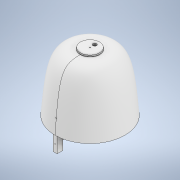
# Autodesk Inventor part: EnclosingRevolver
Saved by Autodesk Inventor 2021.1 (Build 251245010, 245A)
## iProperties
Created: 2023-07-02
Part Number: EnclosingRevolver
Material: ABS Plastic
Document SubType Name: Modeling
Designer: Drake
Density: 1.06 g/cm^3
Appearance: Smooth - White
Author: Drake
Autodesk Inventor part; units mm, degrees
ref_plane "XZ Plane" through (0, 0, 0) normal (0, 1, 0) x (-1, 0, 0)
sketch "Sketch1" plane through (0, 0, 0) normal (0, 1, 0) x (-1, 0, 0)
  circle A0 centre (0, 0) radius 1
  circle A1 centre (0, 0) radius 25
  dimension "d0" = 2
  dimension "d1" = 50
  constraints: 2 centre point, 2 coincident
  measures "d0" diameter of A0
  measures "d1" diameter of A1
extrude "Extrusion1" add sketch "Sketch1" along normal blind 3.7
ref_plane "Work Plane2" through (-25, 0, 0) normal (1, 0, 0) x (0, 1, 0)
ref_plane "Work Plane1" through (25, 0, 0) normal (1, 0, 0) x (0, 1, 0)
sketch "Sketch3" plane through (0, 0, 0) normal (1, 0, 0) x (0, 1, 0)
  line L0 (0, 25.8902) -> (0, 82.1004) construction
  line L1 (0, 82.1004) -> (-19.2329, 82.1004) construction
  line L2 (-19.2329, 82.1004) -> (-150.2459, 92.0453) construction
  line L3 (-150.2459, 92.0453) -> (-151.1107, 92.0453) construction
  spline S0 degree 4 poles (0, 25.8902) (0, 82.1004) (-19.2329, 82.1004) (-150.2459, 92.0453) (-151.1107, 92.0453) knots 1 1 1 1 1 2 2 2 2 2
  line L4 (0, -25) -> (0, 25) projected
  line L5 (-151.1107, 92.0453) -> (-151.1107, 77.0453)
  line L6 (-151.1107, 77.0453) -> (-80.8125, 71.4468) construction
  line L7 (-80.8125, 71.4468) -> (-20.5383, 53.8321) construction
  line L8 (-20.5383, 53.8321) -> (-22.6717, 53.8321) construction
  line L9 (-22.6717, 53.8321) -> (-15, 0) construction
  spline S1 degree 4 poles (-151.1107, 77.0453) (-80.8125, 71.4468) (-20.5383, 53.8321) (-22.6717, 53.8321) (-15, 0) knots 1 1 1 1 1 2 2 2 2 2
  line L10 (0, 25) -> (0, 0)
  line L11 (0, 25) -> (0, 0)
  line L12 (-15, -28.9058) -> (-15, -27.5917)
  line L13 (0, 25.8902) -> (0, -27.5917)
  line L14 (-15, 0) -> (0, 0)
  dimension "d9" = 15
  dimension "d10" = 15
  constraints: 12 end point, 3 horizontal, 2 point on line, 2 vertical, 1 collinear, 1 parallel, 6 other
  measures "d9" distance of L10.end L9.end
  measures "d10" distance of L3.end L5.end
revolve "Revolution1" add sketch "Sketch3" angle 360 about axis through (0, -15, 0) along (0, -1, 0)
mirror "Mirror1" about plane through (0, 0, 0) normal (0, 0, 1) of "Revolution1"
ref_plane "Work Plane3" through (0, 0, 92.0455) normal (0, 0, 1) x (1, 0, 0)
sketch "Sketch4" plane through (0, 0, 92.0455) normal (0, 0, 1) x (1, 0, 0)
  line L0 (-92.0453, -151.1107) -> (92.0453, -151.1107) projected
  line L1 (-92.0453, -151.1107) -> (-92.0453, -139.1107)
  line L2 (-92.0453, -151.1107) -> (-92.0453, -118.1107)
  line L3 (-92.0453, -118.1107) -> (-92.0453, -113.1107)
  line L4 (-92.0453, -113.1107) -> (0, -113.1107)
  point P0 (0, 0)
  point P1 (0, -151.1107)
  dimension "motorwidth" = 12
  dimension "motorlength" = 33
  dimension "allowance" = 5
  constraints: 8 end point, 3 vertical, 1 coincident, 1 perpendicular
  measures "motorwidth" distance of L0.start L1.end
  measures "motorlength" distance of L0.start L2.end
  measures "allowance" distance of L2.end L3.end
hole "Hole1" at (0, -113.1107, 92.0455) direction (0, 0, -1) diameter 3 end through all
thread "Thread1" size "M3x0.5" class "6H" standard "ANSI Metric M Profile" full length
sketch "Sketch5" plane through (0, 3.7, 0) normal (0, 1, 0) x (1, 0, 0)
  point P0 (0, 0)
  point P1 (0.766, -0.6428)
hole "Hole2" at (0.766, 3.7, 0.6428) direction (0, -1, 0) diameter 2 end through all
sketch "Sketch6" plane through (0, -151.1107, 0) normal (0, -1, 0) x (1, 0, 0)
  line L0 (-4.9974, -76.883) -> (-4.9974, -91.9095)
  circle A0 centre (0, 0) radius 92.0453 projected
  line L1 (4.9974, -91.9095) -> (4.9974, -76.883)
  circle A1 centre (0, 0) radius 77.0453
  point P0 (0, 77.0453)
  point P1 (0, 92.0453)
  constraints: 4 end point, 2 point on circle, 1 coincident, 1 parallel, 1 vertical, 3 other
extrude "Extrusion2" add sketch "Sketch6" along normal blind 40 contours A1 L1 A0 L0 picked at (3.8872, -81.9399)
mirror "Mirror2" about plane through (0, 0, 0) normal (0, 0, 1) of "Extrusion2"
sketch "Sketch7" plane through (0, 0, 92.0455) normal (0, 0, 1) x (1, 0, 0)
  line L0 (0, -151.1107) -> (4.9974, -151.1107) projected
  line L1 (0, -151.1107) -> (0, -191.1107)
  line L2 (-4.9974, -191.1107) -> (4.9974, -191.1107) projected
  circle A0 centre (0, -171.1107) radius 0.95
  point P0 (0, 0)
  dimension "d37" = 1.9
  constraints: 2 end point, 2 midpoint, 1 centre point
  measures "d37" diameter of A0
extrude "Extrusion3" add sketch "Sketch7" against normal blind 25
sketch "Sketch8" plane through (0, 3.7, 0) normal (0, 1, 0) x (1, 0, 0)
  arc A0 (0.9397, 0.342) -> (-0.1736, -0.9848) centre (0, 0) ccw construction
  line L0 (0, 0) -> (0, 25) construction
  circle A1 centre (0, 0) radius 25 construction
  circle A2 centre (0, 12.5) radius 5
  dimension "d40" = 10
  constraints: 2 end point, 1 centre point, 1 midpoint, 1 vertical, 1 vertical alignment, 1 other
  measures "d40" diameter of A2
extrude "Extrusion4" cut sketch "Sketch8" against normal through all
mirror "Mirror3" about plane through (0, 0, 0) normal (0, 0, 1) of "Extrusion3"
body "Solid1"
